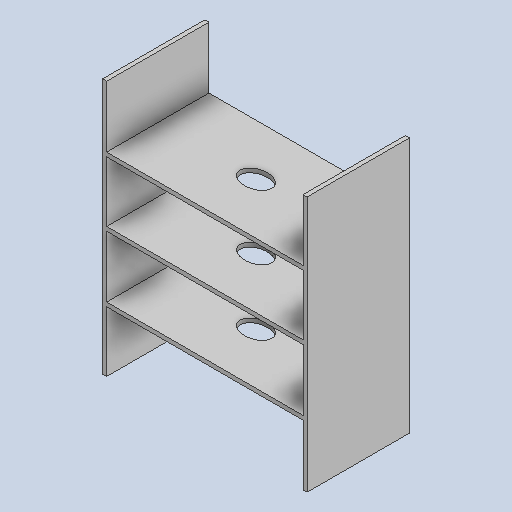
# Autodesk Inventor part: ребра для шкафа
Saved by Autodesk Inventor 2023.1 (Build 271208000, 208)
## iProperties
Created: 2024-11-21
Part Number: ребра для шкафа
Material: Типовые
Document SubType Name: Modeling
Designer: DELL
Density: 1 g/cm^3
Appearance: По умолчанию
Author: DELL
Autodesk Inventor part; units mm, degrees
ref_plane "YZ Plane" through (0, 0, 0) normal (1, 0, 0) x (0, 1, 0)
ref_plane "XZ Plane" through (0, 0, 0) normal (0, 1, 0) x (-1, 0, 0)
ref_plane "XY Plane" through (0, 0, 0) normal (0, 0, 1) x (1, 0, 0)
sketch "Эскиз1" plane through (0, 0, 0) normal (0, 0, 1) x (1, 0, 0)
  line L0 (0, 0) -> (200, 0) construction
  line L1 (10.5713, 250) -> (75.6527, 250) construction
  line L2 (98, 0) -> (102, 0) construction
  line L3 (102, 0) -> (102, 250) construction
  line L4 (98, 250) -> (102, 250) construction
  line L5 (98, 0) -> (98, 250) construction
  line L6 (98, 250) -> (102, 0) construction
  line L7 (0, 127) -> (200, 127)
  line L8 (200, 127) -> (200, 123)
  line L9 (200, 123) -> (0, 123)
  line L10 (0, 123) -> (0, 127)
  line L11 (0, 127) -> (200, 123) construction
  line L12 (200, 127) -> (0, 123) construction
  line L13 (0, 186) -> (200, 186)
  line L14 (200, 186) -> (200, 190)
  line L15 (200, 190) -> (0, 190)
  line L16 (0, 190) -> (0, 186)
  line L17 (0, 0) -> (4, 0)
  line L18 (4, 0) -> (4, 250)
  line L19 (4, 250) -> (0, 250)
  line L20 (0, 250) -> (0, 0)
  line L21 (200, 0) -> (196, 0)
  line L22 (196, 0) -> (196, 250)
  line L23 (196, 250) -> (200, 250)
  line L24 (200, 250) -> (200, 0)
  line L25 (0, 59) -> (200, 59)
  line L26 (200, 59) -> (200, 63)
  line L27 (200, 63) -> (0, 63)
  line L28 (0, 63) -> (0, 59)
  arc A0 (193.3786, 241.9343) -> (189.4287, 250) centre (189.4287, 245) ccw projected
  arc A1 (10.5713, 250) -> (6.6214, 241.9343) centre (10.5713, 245) ccw projected
  arc A2 (0, 0) -> (6.6214, 241.9343) centre (-144.0414, 125) ccw projected
  arc A3 (193.3786, 241.9343) -> (200, 0) centre (344.0414, 125) ccw projected
  arc A4 (78.2507, 248.5) -> (75.6527, 250) centre (75.6527, 247) ccw projected
  line L29 (124.3473, 250) -> (189.4287, 250) projected
  arc A5 (124.3473, 250) -> (121.7493, 248.5) centre (124.3473, 247) ccw projected
  line L30 (121.7493, 248.5) -> (112.751, 232.9146) projected
  arc A6 (108.4209, 230.4146) -> (112.751, 232.9146) centre (108.4209, 235.4146) ccw projected
  line L31 (108.4209, 230.4146) -> (91.5791, 230.4146) projected
  arc A7 (87.249, 232.9146) -> (91.5791, 230.4146) centre (91.5791, 235.4146) ccw projected
  line L32 (87.249, 232.9146) -> (78.2507, 248.5) projected
  point P0 (100, 125)
  point P1 (4, 186)
  point P2 (196, 186)
  point P3 (196, 127)
  point P4 (4, 127)
  point P5 (0, 186)
  point P6 (4, 123)
  point P7 (196, 123)
  point P8 (196, 190)
  point P9 (4, 190)
  point P10 (0, 190)
  point P11 (196, 63)
  point P12 (4, 63)
  point P13 (4, 59)
  point P14 (196, 59)
  dimension "d0" = 200
  dimension "d1" = 4
  dimension "d2" = 200
  dimension "d3" = 4
  dimension "d4" = 4
  dimension "d5" = 250
  dimension "d6" = 4
  dimension "d7" = 250
  dimension "d10" = 60
  dimension "d11" = 200
  dimension "d12" = 4
  dimension "d13" = 60
  constraints: 46 end point, 10 parallel, 5 horizontal, 5 perpendicular, 3 midpoint, 1 point on line
  measures "d0" distance of L8.end L9.end
  measures "d1" distance of L7.end L8.end
  measures "d2" distance of L14.end L15.end
  measures "d3" distance of L13.end L14.end
  measures "d4" distance of L19.end L18.end
  measures "d5" distance of L18.end L17.end
  measures "d6" distance of L22.end L23.end
  measures "d7" distance of L21.end L22.end
  measures "d10" distance between parallel lines of L1 L15
  measures "d11" distance of L27.end L26.end
  measures "d12" distance of L26.end L25.end
  measures "d13" distance between parallel lines of L9 L27
extrude "Выдавливание1" add sketch "Эскиз1" along normal mid plane 100 contours L20 L13 L18 L7 | L7 L18 L9 L10 | L7 A2 L9 L18 | L9 L18 L27 L20 | L16 L15 L18 L13 | L7 A3 L9 A2 | L18 L15 A2 L13 | L27 L18 L25 L20 | L20 L19 L18 L15 | L7 L22 L9 A3 | A2 L15 A3 L13 | L27 A2 L25 L18 | L25 L18 A2 L20 | L22 L13 L24 L7 | L7 L8 L9 L22 | A3 L15 L22 L13 | L27 A3 L25 A2 | A2 L18 L17 | L9 L24 L27 L22 | L22 L15 L14 L13 | L27 L22 L25 A3 | L27 L24 L25 L22 | L22 L23 L24 L15 | L25 L24 A3 L22 | A3 L21 L22
sketch "Эскиз2" plane through (4, 190, 50) normal (0, 1, 0) x (1, 0, 0)
  line L0 (196, 100) -> (196, 0) projected
  line L1 (-4, 0) -> (196, 100) construction
  ellipse E0 centre (96, 50) end of major axis (111.5174, 50) minor radius 11
  point P0 (-4, 50)
  dimension "d16" = 11
  constraints: 2 end point, 1 centre point, 1 midpoint, 1 other
extrude "Выдавливание2" cut sketch "Эскиз2" against normal blind 300
